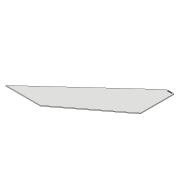
# Autodesk Inventor part: OuterHCALtile12
Saved by Autodesk Inventor 2018 (Build 220112000, 112)
## iProperties
Created: 2017-04-19
Part Number: OuterHCALtile12
Material: ABS Plastic
Document SubType Name: Modeling
Designer: sawaiz
Density: 1.06 g/cm^3
Appearance: Smooth - White
Author: sawaiz
Autodesk Inventor part; units mm, degrees
ref_plane "YZ Plane" through (0, 0, 0) normal (1, 0, 0) x (0, 1, 0)
ref_plane "XZ Plane" through (0, 0, 0) normal (0, 1, 0) x (-1, 0, 0)
ref_plane "XY Plane" through (0, 0, 0) normal (0, 0, 1) x (1, 0, 0)
sketch "Sketch1" plane through (0, 0, 0) normal (0, 1, 0) x (-1, 0, 0)
  line L0 (827.5224, 697.4) -> (514.8224, 697.4)
  line L1 (514.8224, 697.4) -> (0, 304.5)
  line L2 (0, 0) -> (65.6433, 0)
  line L3 (65.6433, 0) -> (827.5224, 697.4)
  line L4 (827.5224, 697.4) -> (827.5224, 0) construction
  line L5 (0, 304.5) -> (0, 691.3725) construction
  line L6 (0, 304.5) -> (0, 0)
  dimension "d0" = 312.7
  dimension "d2" = 697.4
  dimension "d4" = 52.65
  dimension "d5" = 47.53
  dimension "d8" = 304.5
  constraints: 14 end point, 2 vertical, 1 coincident, 1 horizontal, 1 parallel, 1 perpendicular, 1 point on line
  measures "d0" distance of L0.start L0.end
  measures "d2" distance between parallel lines of L0 L2
  measures "d4" angle of L1 L5
  measures "d5" angle of L4 L3
  measures "d8" distance of L1.end L2.start
extrude "Extrusion1" add sketch "Sketch1" along normal mid plane 7
sketch "Sketch2" plane through (0, 3.5, 0) normal (0, 1, 0) x (1, 0, 0)
  line L0 (-827.5224, -697.4) -> (-514.8224, -697.4) projected
  line L1 (-514.8224, -697.4) -> (0, -304.5) projected
  line L2 (0, 0) -> (-65.6433, 0) projected
  line L3 (-65.6433, 0) -> (-827.5224, -697.4) projected
  line L4 (0, 0) -> (-65.6433, 0) projected
  line L5 (-49.7774, 0) -> (-52.2024, -9.05)
  line L6 (-52.2024, -9.05) -> (-11.2524, -9.05)
  line L7 (-11.2524, -9.05) -> (-13.6773, 0)
  line L8 (-22.2224, -9.05) -> (-22.2224, 0) construction
  line L9 (-49.7774, 0) -> (-13.6773, 0)
  line L10 (0, -304.5) -> (0, 0) projected
  dimension "d9" = 75
  dimension "d10" = 75
  dimension "d11" = 9.05
  dimension "d12" = 10.97
  dimension "d13" = 805.3
  dimension "d14" = 40.95
  constraints: 10 end point, 2 horizontal, 1 perpendicular, 1 point on line, 4 other
  measures "d9" angle of L2 L7
  measures "d10" angle of L5 L2
  measures "d11" distance between parallel lines of L2 L6
  measures "d12" distance from line of L8 L6.end
  measures "d13" distance from line of L0.start L8
  measures "d14" distance of L5.end L6.end
extrude "Extrusion2" cut sketch "Sketch2" against normal through all contours L2 L7 L6 L5
fillet "Fillet1" radius 1 2 edges at (-11.2524, 0, 9.05) (-52.2024, 0, 9.05)
sketch "Sketch3" plane through (0, 3.5, 0) normal (0, 1, 0) x (1, 0, 0)
  line L0 (-51.8651, -7.7912) -> (-49.7774, 0) projected
  arc A0 (-51.8651, -7.7912) -> (-50.8991, -9.05) centre (-50.8991, -8.05) ccw projected
  line L1 (-12.5556, -9.05) -> (-50.8991, -9.05) projected
  arc A1 (-12.5556, -9.05) -> (-11.5897, -7.7912) centre (-12.5556, -8.05) ccw projected
  line L2 (-13.6773, 0) -> (-11.5897, -7.7912) projected
  line L3 (-49.7774, 0) -> (-65.6433, 0) projected
  line L4 (-49.7774, 0) -> (-49.7774, 1)
  line L5 (-49.7774, 1) -> (-13.6773, 1)
  line L6 (-11.5897, -7.7912) -> (-13.6773, 0) projected
  line L7 (-13.6773, 1) -> (-13.6773, 0)
  point P0 (0, 0)
  dimension "d18" = 1
  constraints: 6 end point, 1 horizontal, 1 perpendicular, 1 vertical
  measures "d18" distance of L0.end L4.end
extrude "Extrusion3" add sketch "Sketch3" against normal up to surface (7 mm away) separate body
equation "\"d0\" = botWidth"
equation "\"d2\" = height"
equation "\"d4\" = rightAngle"
equation "\"d5\" = leftAngle"
equation "\"d8\" = sideFlat"
equation "\"d13\" = dovetailDistance"
equation "\"height\" = 697.4"
equation "\"botWidth\" = 312.7"
equation "\"leftAngle\" = 47.53deg"
equation "\"rightAngle\" = 52.65deg"
equation "\"sideFlat\" = 304.5"
equation "\"dovetailDistance\" = 805.3"
body "Solid1"
body "Solid2"
